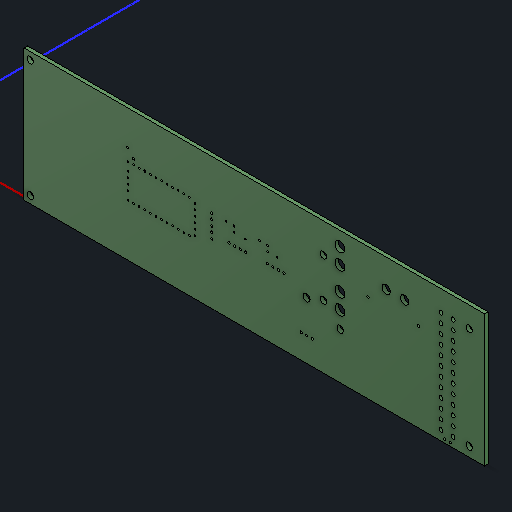
# Autodesk Inventor part: Omnibot_battery_module.brdКонтур
Saved by Autodesk Inventor 2025 (Build 290162000, 162)
## iProperties
Created: 2024-08-13
Part Number: Omnibot_battery_module.brdКонтур
Material: Типовые
Document SubType Name: Modeling
Designer: IvanPetrov
Density: 1 g/cm^3
Appearance: Контур панели
Author: IvanPetrov
Autodesk Inventor part; units mm, degrees
ref_plane "YZ Plane" through (0, 0, 0) normal (1, 0, 0) x (0, 1, 0)
ref_plane "XZ Plane" through (0, 0, 0) normal (0, 1, 0) x (-1, 0, 0)
ref_plane "XY Plane" through (0, 0, 0) normal (0, 0, 1) x (1, 0, 0)
sketch "Эскиз1" plane through (0, 0, 0) normal (0, 0, 1) x (1, 0, 0)
  line L0 (262.54, 30) -> (53, 30)
  line L1 (53, 30) -> (53, -30)
  line L2 (53, -30) -> (262.54, -30)
  line L3 (262.54, -30) -> (262.54, 30)
  circle A0 centre (146.3, -0.13) radius 0.51
  circle A1 centre (148.84, -0.13) radius 0.51
  circle A2 centre (151.38, -0.13) radius 0.51
  circle A3 centre (153.92, -0.13) radius 0.51
  circle A4 centre (171.32, 0.38) radius 0.51
  circle A5 centre (168.78, 0.38) radius 0.51
  circle A6 centre (166.24, 0.38) radius 0.51
  circle A7 centre (163.7, 0.38) radius 0.51
  circle A8 centre (196.72, 5.76) radius 2.275
  circle A9 centre (196.72, -1.44) radius 2.275
  circle A10 centre (196.72, 23.54) radius 2.275
  circle A11 centre (196.72, 16.34) radius 2.275
  circle A12 centre (217.81, 17.27) radius 1.905
  circle A13 centre (226.15, 17.27) radius 1.905
  circle A14 centre (248.25, 20.58) radius 0.9
  circle A15 centre (248.25, 16.38) radius 0.9
  circle A16 centre (248.25, 12.18) radius 0.9
  circle A17 centre (248.25, 7.98) radius 0.9
  circle A18 centre (248.25, 3.78) radius 0.9
  circle A19 centre (248.25, -0.42) radius 0.9
  circle A20 centre (248.25, -4.62) radius 0.9
  circle A21 centre (248.25, -8.82) radius 0.9
  circle A22 centre (248.25, -13.02) radius 0.9
  circle A23 centre (248.25, -17.22) radius 0.9
  circle A24 centre (248.25, -21.42) radius 0.9
  circle A25 centre (248.25, -25.62) radius 0.9
  circle A26 centre (242.75, 20.58) radius 0.9
  circle A27 centre (242.75, 16.38) radius 0.9
  circle A28 centre (242.75, 12.18) radius 0.9
  circle A29 centre (242.75, 7.98) radius 0.9
  circle A30 centre (242.75, 3.78) radius 0.9
  circle A31 centre (242.75, -0.42) radius 0.9
  circle A32 centre (242.75, -4.62) radius 0.9
  circle A33 centre (242.75, -8.82) radius 0.9
  circle A34 centre (242.75, -13.02) radius 0.9
  circle A35 centre (242.75, -17.22) radius 0.9
  circle A36 centre (242.75, -21.42) radius 0.9
  circle A37 centre (242.75, -25.62) radius 0.9
  circle A38 centre (232.41, 10.16) radius 0.51
  circle A39 centre (246.93, -28.49) radius 0.51
  circle A40 centre (244.39, -28.49) radius 0.51
  circle A41 centre (209.55, 10.16) radius 0.51
  circle A42 centre (138.43, -2.54) radius 0.51
  circle A43 centre (138.43, 0) radius 0.51
  circle A44 centre (138.43, 2.54) radius 0.51
  circle A45 centre (138.43, 5.08) radius 0.51
  circle A46 centre (138.43, 7.62) radius 0.51
  circle A47 centre (110.49, 8.89) radius 0.4
  circle A48 centre (113.03, 8.89) radius 0.4
  circle A49 centre (115.57, 8.89) radius 0.4
  circle A50 centre (118.11, 8.89) radius 0.4
  circle A51 centre (100.33, -2.54) radius 0.4
  circle A52 centre (100.33, 0) radius 0.4
  circle A53 centre (100.33, 2.54) radius 0.4
  circle A54 centre (100.33, 5.08) radius 0.4
  circle A55 centre (118.11, -6.35) radius 0.4
  circle A56 centre (115.57, -6.35) radius 0.4
  circle A57 centre (113.03, -6.35) radius 0.4
  circle A58 centre (110.49, -6.35) radius 0.4
  circle A59 centre (107.95, -6.35) radius 0.4
  circle A60 centre (105.41, -6.35) radius 0.4
  circle A61 centre (102.87, -6.35) radius 0.4
  circle A62 centre (100.33, -6.35) radius 0.4
  circle A63 centre (100.33, 8.89) radius 0.4
  circle A64 centre (102.87, 8.89) radius 0.4
  circle A65 centre (105.41, 8.89) radius 0.4
  circle A66 centre (107.95, 8.89) radius 0.4
  circle A67 centre (130.81, 7.62) radius 0.4
  circle A68 centre (125.73, 8.89) radius 0.4
  circle A69 centre (120.65, -6.35) radius 0.4
  circle A70 centre (130.81, -5.08) radius 0.4
  circle A71 centre (130.81, -2.54) radius 0.4
  circle A72 centre (128.27, 8.89) radius 0.4
  circle A73 centre (123.19, 8.89) radius 0.4
  circle A74 centre (123.19, -6.35) radius 0.4
  circle A75 centre (125.73, -6.35) radius 0.4
  circle A76 centre (130.81, 2.54) radius 0.4
  circle A77 centre (128.27, -6.35) radius 0.4
  circle A78 centre (130.81, 5.08) radius 0.4
  circle A79 centre (120.65, 8.89) radius 0.4
  circle A80 centre (130.81, 0) radius 0.4
  circle A81 centre (181.61, -19.05) radius 0.51
  circle A82 centre (184.15, -19.05) radius 0.51
  circle A83 centre (179.07, -19.05) radius 0.51
  circle A84 centre (55.88, 26.67) radius 1.5
  circle A85 centre (55.88, -26.67) radius 1.5
  circle A86 centre (196.85, -8.89) radius 1.5
  circle A87 centre (189.23, 16.51) radius 1.5
  circle A88 centre (189.23, -1.27) radius 1.5
  circle A89 centre (255.5511, -25.6211) radius 1.5
  circle A90 centre (255.5511, 20.5789) radius 1.5
  circle A91 centre (181.61, -4.064) radius 1.651
  circle A92 centre (144.9349, 7.6717) radius 0.4
  circle A93 centre (148.59, 7.62) radius 0.4
  circle A94 centre (148.59, 5.08) radius 0.4
  circle A95 centre (153.67, 5.08) radius 0.4
  circle A96 centre (160.1749, 7.6717) radius 0.4
  circle A97 centre (163.83, 7.62) radius 0.4
  circle A98 centre (163.83, 5.08) radius 0.4
  circle A99 centre (168.1289, 5.0924) radius 0.4
  circle A100 centre (102.87, 11.25) radius 0.5
  circle A101 centre (100.0962, 14.296) radius 0.5
  constraints: 102 centre point, 8 end point
extrude "Omnibot_battery_module.brdКонтур" add sketch "Эскиз1" along normal blind 1.6
